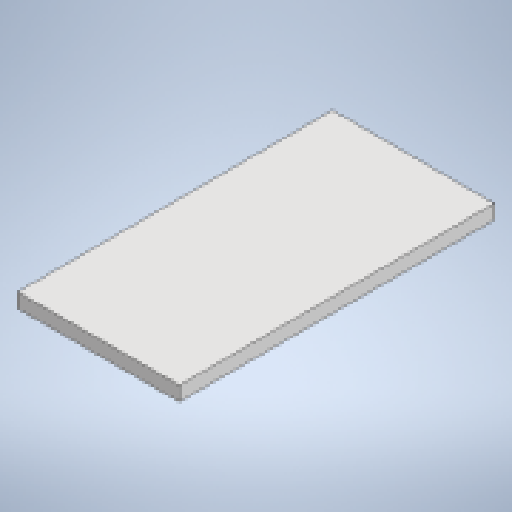
# Autodesk Inventor part: Lateral trasero
Saved by Autodesk Inventor 2024 (Build 280153000, 153)
## iProperties
Created: 2025-03-02
Part Number: Lateral trasero
Material: Genérico
Document SubType Name: Modeling
Designer: sergi
Density: 1 g/cm^3
Appearance: Valor por defecto
Author: sergi
Autodesk Inventor part; units mm, degrees
ref_plane "YZ Plane" through (0, 0, 0) normal (1, 0, 0) x (0, 1, 0)
ref_plane "XZ Plane" through (0, 0, 0) normal (0, 1, 0) x (-1, 0, 0)
ref_plane "Plano de trabajo2" through (33.88, 0, 75) normal (-1, 0, 0) x (0, 0, 1)
sketch "Boceto2" plane through (0, 0, 0) normal (1, 0, 0) x (0, 1, 0)
  line L0 (0, 0) -> (3, 0)
  line L1 (3, 0) -> (3, 78)
  line L2 (3, 78) -> (0, 78)
  line L3 (0, 78) -> (0, 0)
  dimension "d4" = 3
  dimension "d5" = 78
  constraints: 8 end point, 2 parallel, 1 horizontal, 1 perpendicular
  measures "d4" distance of L2.end L1.end
  measures "d5" distance of L1.end L0.end
extrude "Extrusión2" add sketch "Boceto2" along normal up to surface (33.88 mm away)
sketch "Boceto3" plane through (0, 3, 78) normal (0, 1, 0) x (1, 0, 0)
  circle A0 centre (3, 3) radius 2.1 projected
  circle A1 centre (30.88, 3) radius 2.1 projected
  circle A2 centre (3, 75) radius 2.1 projected
  circle A3 centre (28.88, 75) radius 2.1 projected
  point P0 (0, 78)
hole "Agujero1" at (3, 3, 75) at (30.88, 3, 75) at (3, 3, 3) at (28.88, 3, 3) direction (0, -1, 0) diameter 3 depth 5
